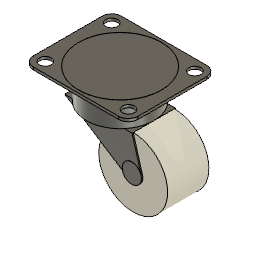
Caster (Autodesk Fusion 360 design; units mm, degrees)
part number: 2026-02-05-15-28-46-463
Autodesk Fusion 360 part; units mm, degrees
sketch "Sketch1" plane through (0, 0, 0) normal (0, 0, 1) x (1, 0, 0)
  circle A0 centre (-15.1, -12.05) radius 2.15
  circle A1 centre (15.1, -12.05) radius 2.15
  circle A2 centre (-15.1, 12.05) radius 2.15
  circle A3 centre (15.1, 12.05) radius 2.15
  line L0 (-15.5, 16) -> (15.5, 16)
  line L1 (19, 12.5) -> (19, -12.5)
  line L2 (15.5, -16) -> (-15.5, -16)
  line L3 (-19, -12.5) -> (-19, 12.5)
  line L4 (0, 16) -> (0, -16) construction
  line L5 (-19, 3.9253) -> (19, -34.3215) construction
  line L6 (-15.1, 12.05) -> (15.1, 12.05) construction
  line L7 (15.1, 12.05) -> (15.1, -12.05) construction
  line L8 (15.1, -12.05) -> (-15.1, -12.05) construction
  line L9 (-15.1, -12.05) -> (-15.1, 12.05) construction
  circle A4 centre (0, 0) radius 15
  arc A5 (-15.5, 16) -> (-19, 12.5) centre (-15.5, 12.5) ccw
  arc A6 (-19, -12.5) -> (-15.5, -16) centre (-15.5, -12.5) ccw
  arc A7 (15.5, -16) -> (19, -12.5) centre (15.5, -12.5) ccw
  arc A8 (19, 12.5) -> (15.5, 16) centre (15.5, 12.5) ccw
  line L10 (-19, 0) -> (19, 0) construction
  point P0 (-19, 16)
  point P1 (19, 16)
  point P2 (-19, -16)
  point P3 (0, 12.05)
  point P4 (-15.1, 0)
  dimension "d1" = 4.3
  dimension "d4" = 30.2
  dimension "d5" = 24.1
  dimension "d6" = 38
  dimension "d7" = 32
  dimension "d8" = 30
  dimension "d9" = 3.5
  constraint horizontal L0
  constraint vertical L1
  constraint horizontal L2
  constraint vertical L3
  constraint midpoint L4 A4.centre
  constraint horizontal L6
  constraint vertical L7
  constraint horizontal L8
  constraint vertical L9
  constraint coincident A1.centre L7.end
  constraint coincident A2.centre L6.start
  constraint midpoint L6 P3
  constraint midpoint L9 P4
  constraint coincident L5 P4
  constraint coincident L4 P3
  constraint coincident A4.centre origin
  constraint coincident L0 L4.start
  constraint coincident L3 L5.start
  constraint coincident P0 L0
  constraint coincident P0 L3
  constraint tangent L0 A5
  constraint tangent L3 A5
  constraint coincident L2 L4.end
  constraint coincident P2 L2
  constraint coincident P2 L3
  constraint tangent L2 A6
  constraint tangent L3 A6
  constraint equal A5 A6
  constraint coincident L1 L5.end
  constraint tangent L1 A7
  constraint tangent L2 A7
  constraint equal A5 A7
  constraint coincident P1 L0
  constraint coincident P1 L1
  constraint tangent L0 A8
  constraint tangent L1 A8
  constraint equal A5 A8
  constraint perpendicular L0 L4
  constraint midpoint L3 L10.start
  constraint midpoint L1 L10.end
  constraint coincident P4 L10
  constraint midpoint L10 A4.centre
  measures "d1" diameter of A0
  measures "d6" distance of P0 P1
  measures "d7" distance of P0 P2
  measures "d8" diameter of A4
  measures "d9" radius of A5
extrude "Extrude1" add sketch "Sketch1" along normal blind 1 makes body 1
extrude "Extrude2" add sketch "Sketch1" along normal blind 0.95 contours A4 bodies 1
sketch "Sketch2" plane through (0, 0, 0) normal (0, 0, 1) x (1, 0, 0)
  circle A0 centre (-15.1, -12.05) radius 2.15
  circle A1 centre (15.1, 12.05) radius 2.15
  circle A2 centre (15.1, -12.05) radius 2.15
  circle A3 centre (-15.1, 12.05) radius 2.15
  arc A4 (15.5, -16) -> (19, -12.5) centre (15.5, -12.5) ccw
  line L0 (15.5, -16) -> (-15.5, -16)
  arc A5 (-19, -12.5) -> (-15.5, -16) centre (-15.5, -12.5) ccw
  line L1 (-19, -12.5) -> (-19, 12.5)
  arc A6 (-15.5, 16) -> (-19, 12.5) centre (-15.5, 12.5) ccw
  line L2 (-15.5, 16) -> (15.5, 16)
  arc A7 (19, 12.5) -> (15.5, 16) centre (15.5, 12.5) ccw
  line L3 (19, 12.5) -> (19, -12.5)
  circle A8 centre (0, 0) radius 12.25
  dimension "d14" = 24.5
  constraint coincident A8.centre origin
  measures "d14" diameter of A8
extrude "Extrude3" add sketch "Sketch2" against normal blind 10 contours A8 bodies 1
ref_plane "WorkPlane1" through (0, 0, 0.5) normal (0, -1, 0) x (1, 0, 0)
sketch "Sketch3" plane through (0, 0, 0) normal (0, -1, 0) x (-1, 0, 0)
  line L0 (12.25, 10) -> (-12.25, 10)
  line L1 (-12.25, 0) -> (12.25, 0)
  circle A0 centre (-12.25, 22.5) radius 12.5
  circle A1 centre (-12.25, 22.5) radius 3.5
  line L2 (-15.61, 21.52) -> (-12.25, 10)
  line L3 (-15.61, 21.52) -> (-8.89, 23.48) construction
  line L4 (-8.89, 23.48) -> (12.25, 10)
  dimension "d17" = 25
  dimension "d18" = 7
  dimension "d19" = 12
  constraint vertical L0.end A0.centre
  constraint coincident L0.end A0
  constraint concentric A0 A1
  constraint coincident A1 L2.start
  constraint coincident L0.end L2.end
  constraint coincident A1 L3.end
  constraint perpendicular L2 L3
  constraint coincident L0.start L4.end
  measures "d17" diameter of A0
  measures "d18" diameter of A1
  measures "d19" distance of L2.start L0.end
extrude "Extrude4" add sketch "Sketch3" along normal mid plane 15 separate body contours A0 A1 L2 L4 | A0 A1 L2 L4 | A1 makes body 2
extrude "Extrude5" add sketch "Sketch3" along normal mid plane 16 contours A1 bodies 2
extrude "Extrude6" add sketch "Sketch3" along normal mid plane 15.8 contours L0 A0 L4 | A0 A1 L2 L4 picked at (-3.6072, 18.6024) bodies 1 2
equation "d4 = 25.9 mm + 4.3 mm"
equation "d5 = 19.8 mm + 4.3 mm"
equation "d20 = ( 15 / 2 ) * 1 mm"
